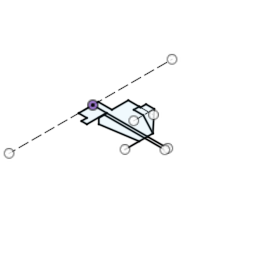
magnet catch v2 (Autodesk Fusion 360 design; units mm, degrees)
Autodesk Fusion 360 part; units mm, degrees
sketch "cross section" plane through (0, 0, 0) normal (0, 1, 0) x (1, 0, 0)
  line L0 (0, 0) -> (13.7411, 0)
  line L1 (2.5, 0) -> (2.5, -3.5899)
  line L2 (2.5, -3.5899) -> (1.5, -3.5899)
  line L3 (1.5, -3.5899) -> (1.5, -2.5899)
  line L4 (1.5, -2.5899) -> (0, -2.5899)
  line L5 (0, 0) -> (0, -15.3536) construction
  line L6 (0, 0) -> (0, 14.5137) construction
  line L7 (2.6, 0) -> (2.6, -1.5)
  line L8 (2.6, -1.5) -> (3.5899, -2.4899)
  line L9 (2.6, -0.5) -> (13.7041, -0.5)
  line L10 (0, 1) -> (2.5, 1)
  line L11 (2.5, 1) -> (2.5, 4)
  line L12 (2.5, 4) -> (4.5, 4)
  line L13 (4.5, 4) -> (7.1203, 4) construction
  line L14 (4.5, 4) -> (4.5, 3)
  line L15 (10, 1) -> (10, 0)
  line L16 (10, 0) -> (10, -4.1086)
  line L17 (3.5899, -2.4899) -> (10, -1.5)
  line L18 (0, 1) -> (0, -2.5899)
  line L19 (4.5, 4) -> (4.75, 4)
  line L20 (4.75, 4) -> (4.75, 5)
  line L21 (4.75, 5) -> (6.25, 5)
  line L22 (6.25, 5) -> (10, 1)
  line L23 (6.25, 5) -> (6.25, 1.2504) construction
  line L24 (4.5, 3) -> (6.25, 3)
  line L25 (6.25, 3) -> (10, 1)
  dimension "d1" = 1
  dimension "d2" = 1
  dimension "d3" = 2.5
  dimension "d4" = 135
  dimension "d5" = 1.4
  dimension "d6" = 0.1
  dimension "d7" = 0.5
  dimension "d8" = 1
  dimension "d9" = 0.1
  dimension "d10" = 2.5
  dimension "d11" = 3
  dimension "d12" = 2
  dimension "d14" = 1
  dimension "d15" = 1
  dimension "d16" = 1
  dimension "d17" = 10
  dimension "d18" = 1
  dimension "d19" = 0.25
  dimension "d20" = 1
  dimension "d21" = 1.5
  constraint coincident L0.start L5.start
  constraint horizontal L0
  constraint coincident L0 L1.start
  constraint perpendicular L0 L1
  constraint perpendicular L1 L2
  constraint perpendicular L2 L3
  constraint perpendicular L3 L4
  constraint perpendicular L0 L5
  constraint perpendicular L0 L6
  constraint coincident L0 L7.start
  constraint perpendicular L0 L7
  constraint coincident L7 L9.start
  constraint perpendicular L7 L9
  constraint coincident L6 L10.start
  constraint perpendicular L6 L10
  constraint perpendicular L10 L11
  constraint perpendicular L11 L12
  constraint horizontal L13
  constraint perpendicular L13 L14
  constraint coincident L0 L15.end
  constraint perpendicular L0 L15
  constraint perpendicular L9 L16
  constraint coincident L16 L17.end
  constraint perpendicular L4 L18
  constraint perpendicular L14 L19
  constraint perpendicular L13 L20
  constraint perpendicular L20 L21
  constraint perpendicular L21 L23
  constraint coincident L23 L24.end
  constraint perpendicular L23 L24
  measures "d1" distance of L1.end L2.end
  measures "d2" distance of L2.end L3.end
  measures "d3" distance of L1 L5
  measures "d4" angle of L7 L8
  measures "d5" distance of L7.end L8.end
  measures "d6" distance of L1 L7
  measures "d7" distance of L0 L9
  measures "d8" distance of L7.end L9
  measures "d9" distance of L4 L8.end
  measures "d10" distance of L10.start L10.end
  measures "d11" distance of L10.end L11.end
  measures "d12" distance of L11.end L12.end
  measures "d14" distance of L12.end L14.end
  measures "d15" distance of L0 L10
  measures "d16" distance of L15.start L15.end
  measures "d17" distance of L6 L15
  measures "d18" distance of L9 L17.end
  measures "d19" distance of L12.end L19.end
  measures "d20" distance of L19.end L20.end
  measures "d21" distance of L20.end L21.end
revolve "Revolve1" add sketch "cross section" angle 360 about axis through (0, 0, 0) along (0, 0, -1) contours L7 L8 L9 L16 L17 makes body 1
revolve "Revolve2" add sketch "cross section" angle 360 about axis through (0, 0, 0) along (0, 0, -1) separate body contours L0 L10 L11 L12 L14 L15 L18 L24 L25 | L0 L1 L2 L3 L4 L18 makes body 2
revolve "Revolve3" add sketch "cross section" angle 360 about axis through (0, 0, 0) along (0, 0, -1) separate body contours L0 L10 L11 L12 L14 L15 L18 L24 L25 | L0 L1 L2 L3 L4 L18 | L14 L19 L20 L21 L22 L24 L25 makes body 3
hidden bodies 1 2 3
named bodies: "magnet catch back", "magnet catch plug", "magnet catch socket"
